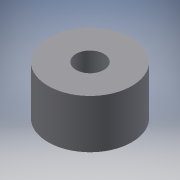
# Autodesk Inventor part: lazy susan bushing
Saved by Autodesk Inventor 2017 (Build 210142000, 142)
## iProperties
Created: 2016-10-04
Part Number: lazy susan bushing
Material: Generic
Document SubType Name: Modeling
Designer: hanso
Density: 1 g/cm^3
Appearance: Default
Author: hanso
Autodesk Inventor part; units mm, degrees
ref_plane "YZ Plane" through (0, 0, 0) normal (1, 0, 0) x (0, 1, 0)
ref_plane "XZ Plane" through (0, 0, 0) normal (0, 1, 0) x (-1, 0, 0)
ref_plane "XY Plane" through (0, 0, 0) normal (0, 0, 1) x (1, 0, 0)
sketch "Sketch1" plane through (0, 0, 0) normal (0, 1, 0) x (-1, 0, 0)
  circle A0 centre (0, 0) radius 9.525
  circle A1 centre (0, 0) radius 3.175
  dimension "d0" = 19.05
  dimension "d1" = 6.35
  constraints: 2 centre point, 2 coincident
  measures "d0" diameter of A0
  measures "d1" diameter of A1
extrude "Extrusion1" add sketch "Sketch1" along normal blind 12.7
sketch "Sketch2" plane through (0, 0, 0) normal (0, -1, 0) x (1, 0, 0)
  circle A0 centre (0, 0) radius 3.175 projected
  circle A1 centre (0, 0) radius 9.525
  constraints: 1 centre point, 1 coincident
extrude "Extrusion2" cut sketch "Sketch2" against normal blind 1.6002
body "Solid1"
